FinAttachment v3 (Autodesk Fusion 360 design; units mm, degrees)
Autodesk Fusion 360 part; units mm, degrees
sketch "Sketch1" plane through (0, 0, 0) normal (0, 1, 0) x (1, 0, 0)
  arc A0 (-9.861, -36.8018) -> (0, -38.1) centre (0, 0) ccw
  line L0 (0, -38.1) -> (0, -48.1)
  line L1 (0, -48.1) -> (-9.861, -36.8018)
  line L2 (0, 0) -> (-9.861, -36.8018) construction
  line L3 (0, -38.1) -> (0, 0) construction
  line L4 (-3.8826, -38.1) -> (9.4481, -38.1) construction
  dimension "d1" = 38.1
  dimension "d2" = 15
  dimension "d3" = 10
  constraint coincident A0.centre L2.start
  constraint tangent A0 L4
  constraint perpendicular L3 L4
  constraint collinear A0.centre A0.end L0.end
  constraint vertical L0
  measures "d1" radius of A0
  measures "d2" angle of L2 L3
  measures "d3" distance of A0.end L0.end
extrude "Extrude1" add sketch "Sketch1" along normal blind 75
equation "d1 = ( 76.20 / 2 ) * 1 mm"
